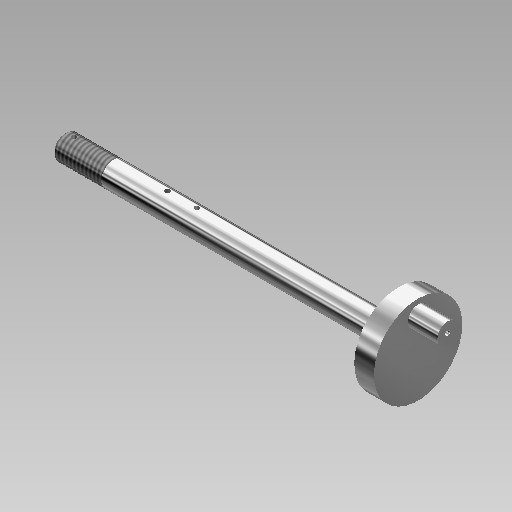
# Autodesk Inventor part: shaft
Saved by Autodesk Inventor 2018.1 (Build 221171000, 171)
## iProperties
Created: 2013-08-27
Part Number: shaft
Material: Generic
Document SubType Name: Modeling
Designer: Konstantin
Density: 1 g/cm^3
Appearance: Default
Mass: 2.41744 g
Surface Area: 19.3881 cm^2
Volume: 2.41744 cm^3
Author: Konstantin
Autodesk Inventor part; units mm, degrees
ref_plane "YZ Plane" through (0, 0, 0) normal (1, 0, 0) x (0, 1, 0)
ref_plane "XZ Plane" through (0, 0, 0) normal (0, 1, 0) x (-1, 0, 0)
ref_plane "XY Plane" through (0, 0, 0) normal (0, 0, 1) x (1, 0, 0)
sketch "Sketch1" plane through (0, 0, 0) normal (0, 0, 1) x (1, 0, 0)
  line L0 (0, 0) -> (72, 0)
  line L1 (68, 2.5) -> (0, 2.5)
  line L2 (0, 2.5) -> (0, 0)
  line L3 (68, 2.5) -> (68, 9)
  line L4 (68, 9) -> (72, 9)
  line L5 (72, 9) -> (72, 0)
  constraints: 12 end point, 3 horizontal, 3 vertical, 2 parallel
revolve "Revolution1" add sketch "Sketch1" angle 360 about axis through (0, 0, 0) along (1, 0, 0)
chamfer "Chamfer1" distance 0.5 angle 45 1 edges at (0, -2.5, 0)
thread "Thread1" size "M5x0.8" class "6g" standard "ISO Metric profile" length 10 offset 58
sketch "Sketch2" plane through (72, 0, 0) normal (1, 0, 0) x (0, 0, -1)
  circle A0 centre (0, 5.9) radius 2.1
  circle A1 centre (0, 5.9) radius 0.5
  constraints: 2 centre point, 1 coincident, 2 other
extrude "Extrusion1" add sketch "Sketch2" along normal blind 6
sketch "Sketch3" plane through (0, 0, 0) normal (0, 1, 0) x (-1, 0, 0)
  circle A0 centre (-2, 0) radius 0.5
  constraints: 1 centre point, 1 other
extrude "Extrusion2" cut sketch "Sketch3" along normal mid plane 10
sketch "Sketch4" plane through (0, 0, 0) normal (0, 1, 0) x (-1, 0, 0)
  circle A0 centre (-27, 0) radius 0.5
  constraints: 1 centre point, 1 other
extrude "Extrusion3" cut sketch "Sketch4" along normal mid plane 10
sketch "Sketch5" plane through (0, 0, 0) normal (0, 1, 0) x (-1, 0, 0)
  circle A0 centre (-21, 0) radius 0.525
  constraints: 1 centre point, 1 other
extrude "Extrusion4" cut sketch "Sketch5" along normal mid plane 10
body "Solid1"
